Autodesk Inventor part; units mm, degrees
(part 3 of 3)
  line L680 (638.3688, 339.2047) -> (638.9016, 338.76)
  line L681 (638.9016, 338.76) -> (639.2596, 338.5571)
  line L682 (639.2596, 338.5571) -> (639.6267, 338.3665)
  line L683 (639.6267, 338.3665) -> (639.8959, 338.2197)
  line L684 (639.8959, 338.2197) -> (640.078, 338.1171)
  line L685 (640.078, 338.1171) -> (640.2676, 338.0095)
  line L686 (640.2676, 338.0095) -> (640.5028, 338.03)
  line L687 (640.5028, 338.03) -> (640.6816, 338.0539)
  line L688 (640.6816, 338.0539) -> (640.8096, 337.8945)
  line L689 (640.8096, 337.8945) -> (640.9312, 337.6444)
  line L690 (640.9312, 337.6444) -> (641.074, 337.467)
  line L691 (641.074, 337.467) -> (641.2513, 337.3173)
  line L692 (641.2513, 337.3173) -> (641.4497, 337.221)
  line L693 (641.4497, 337.221) -> (641.6459, 337.2855)
  line L694 (641.6459, 337.2855) -> (641.7783, 337.4818)
  line L695 (641.7783, 337.4818) -> (641.7901, 337.7652)
  line L696 (641.7901, 337.7652) -> (641.6541, 338.0807)
  line L697 (641.6541, 338.0807) -> (641.4196, 338.3328)
  line L698 (641.4196, 338.3328) -> (641.359, 338.4957)
  line L699 (641.359, 338.4957) -> (641.5219, 338.6755)
  line L700 (641.5219, 338.6755) -> (641.6875, 338.8527)
  line L701 (641.6875, 338.8527) -> (641.8397, 339.012)
  line L702 (641.8397, 339.012) -> (641.9195, 339.164)
  line L703 (641.9195, 339.164) -> (641.91, 339.3267)
  line L704 (641.91, 339.3267) -> (641.8249, 339.4845)
  line L705 (641.8249, 339.4845) -> (641.8179, 339.6062)
  line L706 (641.8179, 339.6062) -> (641.8756, 339.7158)
  line L707 (641.8756, 339.7158) -> (641.9948, 339.8783)
  line L708 (641.9948, 339.8783) -> (642.1243, 340.1092)
  line L709 (642.1243, 340.1092) -> (642.1842, 340.3675)
  line L710 (642.1842, 340.3675) -> (642.1632, 340.876)
  line L711 (642.1632, 340.876) -> (642.4317, 341.3803)
  line L712 (642.4317, 341.3803) -> (643.0116, 341.5945)
  line L713 (643.0116, 341.5945) -> (643.662, 341.6192)
  line L714 (643.662, 341.6192) -> (644.1803, 341.6752)
  line L715 (644.1803, 341.6752) -> (644.6825, 341.7873)
  line L716 (644.6825, 341.7873) -> (645.1009, 341.94)
  line L717 (645.1009, 341.94) -> (645.2923, 342.2013)
  line L718 (645.2923, 342.2013) -> (645.2999, 342.5311)
  line L719 (645.2999, 342.5311) -> (645.1703, 342.8111)
  line L720 (645.1703, 342.8111) -> (645.0727, 343.0529)
  line L721 (645.0727, 343.0529) -> (645.0009, 343.307)
  line L722 (645.0009, 343.307) -> (644.9495, 343.5589)
  line L723 (644.9495, 343.5589) -> (644.9292, 343.8126)
  line L724 (644.9292, 343.8126) -> (644.9075, 344.0655)
  line L725 (644.9075, 344.0655) -> (644.8528, 344.2885)
  line L726 (644.8528, 344.2885) -> (644.7662, 344.4784)
  line L727 (644.7662, 344.4784) -> (644.6518, 344.6546)
  line L728 (644.6518, 344.6546) -> (644.5158, 344.8274)
  line L729 (644.5158, 344.8274) -> (644.4573, 345.0121)
  line L730 (644.4573, 345.0121) -> (644.4937, 345.193)
  line L731 (644.4937, 345.193) -> (644.681, 345.4942)
  line L732 (644.681, 345.4942) -> (645.0696, 345.8439)
  line L733 (645.0696, 345.8439) -> (645.5473, 346.0497)
  line L734 (645.5473, 346.0497) -> (646.292, 346.1333)
  line L735 (646.292, 346.1333) -> (647.2654, 345.9804)
  line L736 (647.2654, 345.9804) -> (648.181, 345.6131)
  line L737 (648.181, 345.6131) -> (649.162, 345.0699)
  line L738 (649.162, 345.0699) -> (650.2162, 344.352)
  line L739 (650.2162, 344.352) -> (651.156, 343.4951)
  line L740 (651.156, 343.4951) -> (651.8587, 342.5889)
  line L741 (651.8587, 342.5889) -> (652.3075, 341.7803)
  line L742 (652.3075, 341.7803) -> (652.6357, 340.9186)
  line L743 (652.6357, 340.9186) -> (652.8597, 339.9664)
  line L744 (652.8597, 339.9664) -> (653.0795, 338.9452)
  line L745 (653.0795, 338.9452) -> (653.2815, 337.921)
  line L746 (653.2815, 337.921) -> (653.4749, 336.6266)
  line L747 (653.4749, 336.6266) -> (653.6329, 334.9303)
  line L748 (653.6329, 334.9303) -> (653.64, 333.2269)
  line L749 (653.64, 333.2269) -> (653.5125, 331.9053)
  line L750 (653.5125, 331.9053) -> (653.4527, 331.1762)
  line L751 (653.4527, 331.1762) -> (653.4097, 330.445)
  line L752 (653.4097, 330.445) -> (653.3768, 329.9973)
  line L753 (653.3768, 329.9973) -> (653.341, 329.9847)
  line L754 (653.341, 329.9847) -> (653.3006, 329.9705)
  line L755 (653.3006, 329.9705) -> (653.2343, 330.0785)
  line L756 (653.2343, 330.0785) -> (653.0864, 330.3682)
  line L757 (653.0864, 330.3682) -> (652.9397, 330.6585)
  line L758 (652.9397, 330.6585) -> (652.5578, 331.4365)
  line L759 (652.5578, 331.4365) -> (651.7302, 332.977)
  line L760 (651.7302, 332.977) -> (650.7272, 334.4004)
  line L761 (650.7272, 334.4004) -> (649.6787, 335.4361)
  line L762 (649.6787, 335.4361) -> (648.9013, 336.0163)
  line L763 (648.9013, 336.0163) -> (648.0503, 336.4816)
  line L764 (648.0503, 336.4816) -> (647.2286, 336.7737)
  line L765 (647.2286, 336.7737) -> (646.5919, 336.9521)
  line L766 (646.5919, 336.9521) -> (645.9486, 337.0788)
  line L767 (645.9486, 337.0788) -> (645.3737, 337.118)
  line L768 (645.3737, 337.118) -> (644.935, 337.0846)
  line L769 (644.935, 337.0846) -> (644.4965, 337.0158)
  line L770 (644.4965, 337.0158) -> (644.0896, 336.9396)
  line L771 (644.0896, 336.9396) -> (643.7371, 336.8506)
  line L772 (643.7371, 336.8506) -> (643.3867, 336.7494)
  line L773 (643.3867, 336.7494) -> (642.9684, 336.6283)
  line L774 (642.9684, 336.6283) -> (642.4606, 336.4025)
  line L775 (642.4606, 336.4025) -> (641.9974, 336.1008)
  line L776 (641.9974, 336.1008) -> (641.4154, 335.5958)
  line L777 (641.4154, 335.5958) -> (640.6559, 334.7195)
  line L778 (640.6559, 334.7195) -> (640.0496, 333.7342)
  line L779 (640.0496, 333.7342) -> (639.598, 332.6628)
  line L780 (639.598, 332.6628) -> (639.4033, 331.5928)
  line L781 (639.4033, 331.5928) -> (639.5285, 330.5297)
  line L782 (639.5285, 330.5297) -> (639.9163, 329.6261)
  line L783 (639.9163, 329.6261) -> (640.2591, 329.0578)
  line L784 (640.2591, 329.0578) -> (640.7016, 328.5777)
  line L785 (640.7016, 328.5777) -> (641.3259, 328.2297)
  line L786 (641.3259, 328.2297) -> (642.0543, 327.9898)
  line L787 (642.0543, 327.9898) -> (642.8045, 327.9153)
  line L788 (642.8045, 327.9153) -> (643.4239, 328.0198)
  line L789 (643.4239, 328.0198) -> (643.7234, 328.164)
  line L790 (643.7234, 328.164) -> (644.0036, 328.3597)
  line L791 (644.0036, 328.3597) -> (644.2303, 328.545)
  line L792 (644.2303, 328.545) -> (644.3579, 328.5949)
  line L793 (644.3579, 328.5949) -> (644.4647, 328.5515)
  line L794 (644.4647, 328.5515) -> (644.6078, 328.5483)
  line L795 (644.6078, 328.5483) -> (644.8137, 328.7622)
  line L796 (644.8137, 328.7622) -> (645.0075, 328.9633)
  line L797 (645.0075, 328.9633) -> (645.2007, 329.0779)
  line L798 (645.2007, 329.0779) -> (645.4102, 329.0354)
  line L799 (645.4102, 329.0354) -> (645.6024, 328.9962)
  line L800 (645.6024, 328.9962) -> (645.775, 329.1124)
  line L801 (645.775, 329.1124) -> (645.9143, 329.5669)
  line L802 (645.9143, 329.5669) -> (646.0494, 330.0046)
  line L803 (646.0494, 330.0046) -> (646.1598, 330.3696)
  line L804 (646.1598, 330.3696) -> (646.1419, 330.5458)
  line L805 (646.1419, 330.5458) -> (646.04, 330.6792)
  line L806 (646.04, 330.6792) -> (645.7833, 330.864)
  line L807 (645.7833, 330.864) -> (645.4962, 331.381)
  line L808 (645.4962, 331.381) -> (645.5693, 331.9567)
  line L809 (645.5693, 331.9567) -> (645.9469, 332.3437)
  line L810 (645.9469, 332.3437) -> (646.3957, 332.4185)
  line L811 (646.3957, 332.4185) -> (646.8578, 332.3259)
  line L812 (646.8578, 332.3259) -> (647.1637, 332.0494)
  line L813 (647.1637, 332.0494) -> (647.2902, 331.5479)
  line L814 (647.2902, 331.5479) -> (647.1838, 331.048)
  line L815 (647.1838, 331.048) -> (646.9158, 330.7499)
  line L816 (646.9158, 330.7499) -> (646.8237, 330.6249)
  line L817 (646.8237, 330.6249) -> (646.8245, 330.496)
  line L818 (646.8245, 330.496) -> (646.909, 330.2956)
  line L819 (646.909, 330.2956) -> (647.078, 329.9354)
  line L820 (647.078, 329.9354) -> (647.2514, 329.5773)
  line L821 (647.2514, 329.5773) -> (647.4089, 329.2696)
  line L822 (647.4089, 329.2696) -> (647.5223, 329.1487)
  line L823 (647.5223, 329.1487) -> (647.6603, 329.1508)
  line L824 (647.6603, 329.1508) -> (647.8084, 329.2959)
  line L825 (647.8084, 329.2959) -> (647.9268, 329.3852)
  line L826 (647.9268, 329.3852) -> (648.0544, 329.3725)
  line L827 (648.0544, 329.3725) -> (648.1713, 329.2651)
  line L828 (648.1713, 329.2651) -> (648.2406, 329.2248)
  line L829 (648.2406, 329.2248) -> (648.3206, 329.1923)
  line L830 (648.3206, 329.1923) -> (648.4374, 329.1145)
  line L831 (648.4374, 329.1145) -> (648.6695, 329.026)
  line L832 (648.6695, 329.026) -> (648.8857, 329.0926)
  line L833 (648.8857, 329.0926) -> (649.1375, 329.3402)
  line L834 (649.1375, 329.3402) -> (649.338, 329.6124)
  line L835 (649.338, 329.6124) -> (649.2845, 329.8203)
  line L836 (649.2845, 329.8203) -> (648.9894, 330.1015)
  line L837 (648.9894, 330.1015) -> (648.8461, 330.3743)
  line L838 (648.8461, 330.3743) -> (648.8467, 330.6597)
  line L839 (648.8467, 330.6597) -> (648.9019, 330.9534)
  line L840 (648.9019, 330.9534) -> (649.0437, 331.1526)
  line L841 (649.0437, 331.1526) -> (649.2599, 331.256)
  line L842 (649.2599, 331.256) -> (649.5081, 331.3325)
  line L843 (649.5081, 331.3325) -> (649.7429, 331.4624)
  line L844 (649.7429, 331.4624) -> (649.8689, 331.644)
  line L845 (649.8689, 331.644) -> (649.8709, 331.9244)
  line L846 (649.8709, 331.9244) -> (649.7689, 332.2531)
  line L847 (649.7689, 332.2531) -> (649.5634, 332.4074)
  line L848 (649.5634, 332.4074) -> (649.1862, 332.4392)
  line L849 (649.1862, 332.4392) -> (648.8348, 332.4703)
  line L850 (648.8348, 332.4703) -> (648.6591, 332.6342)
  line L851 (648.6591, 332.6342) -> (648.5396, 332.9759)
  line L852 (648.5396, 332.9759) -> (648.5396, 333.1972)
  line L853 (648.5396, 333.1972) -> (648.5993, 333.4307)
  line L854 (648.5993, 333.4307) -> (648.6908, 333.6545)
  line L855 (648.6908, 333.6545) -> (648.7603, 333.8764)
  line L856 (648.7603, 333.8764) -> (648.7114, 334.0594)
  line L857 (648.7114, 334.0594) -> (648.5368, 334.1793)
  line L858 (648.5368, 334.1793) -> (648.5255, 334.1971)
  line L859 (648.5255, 334.1971) -> (648.4352, 334.2619)
  line L860 (648.4352, 334.2619) -> (648.1296, 334.43)
  line L861 (648.1296, 334.43) -> (647.8956, 334.3619)
  line L862 (647.8956, 334.3619) -> (647.5624, 334.0726)
  line L863 (647.5624, 334.0726) -> (647.1848, 333.9698)
  line L864 (647.1848, 333.9698) -> (646.8096, 334.0976)
  line L865 (646.8096, 334.0976) -> (646.6055, 334.3548)
  line L866 (646.6055, 334.3548) -> (646.5912, 334.3837)
  line L867 (646.5912, 334.3837) -> (646.5764, 334.4123)
  line L868 (646.5764, 334.4123) -> (646.5328, 334.5402)
  line L869 (646.5328, 334.5402) -> (646.36, 334.9153)
  line L870 (646.36, 334.9153) -> (646.1032, 335.0114)
  line L871 (646.1032, 335.0114) -> (645.6643, 334.9395)
  line L872 (645.6643, 334.9395) -> (645.4263, 334.8369)
  line L873 (645.4263, 334.8369) -> (645.3011, 334.6517)
  line L874 (645.3011, 334.6517) -> (645.2925, 334.3663)
  line L875 (645.2925, 334.3663) -> (645.3093, 334.0823)
  line L876 (645.3093, 334.0823) -> (645.2219, 333.8429)
  line L877 (645.2219, 333.8429) -> (644.945, 333.7417)
  line L878 (644.945, 333.7417) -> (644.6953, 333.7646)
  line L879 (644.6953, 333.7646) -> (644.4442, 333.8373)
  line L880 (644.4442, 333.8373) -> (644.2089, 333.9335)
  line L881 (644.2089, 333.9335) -> (644.0187, 333.9855)
  line L882 (644.0187, 333.9855) -> (643.8593, 333.9464)
  line L883 (643.8593, 333.9464) -> (643.7235, 333.7943)
  line L884 (643.7235, 333.7943) -> (643.6129, 333.639)
  line L885 (643.6129, 333.639) -> (643.5021, 333.4846)
  line L886 (643.5021, 333.4846) -> (643.4129, 333.3388)
  line L887 (643.4129, 333.3388) -> (643.4033, 333.2638)
  line L888 (643.4033, 333.2638) -> (643.4201, 333.1782)
  line L889 (643.4201, 333.1782) -> (643.4548, 333.1005)
  line L890 (643.4548, 333.1005) -> (643.5125, 333.014)
  line L891 (643.5125, 333.014) -> (643.5832, 332.9366)
  line L892 (643.5832, 332.9366) -> (643.6908, 332.8603)
  line L893 (643.6908, 332.8603) -> (643.873, 332.6566)
  line L894 (643.873, 332.6566) -> (643.9145, 332.4144)
  line L895 (643.9145, 332.4144) -> (643.8537, 332.1496)
  line L896 (643.8537, 332.1496) -> (643.707, 331.9584)
  line L897 (643.707, 331.9584) -> (643.4973, 331.8541)
  line L898 (643.4973, 331.8541) -> (643.2471, 331.7944)
  line L899 (643.2471, 331.7944) -> (642.9748, 331.7079)
  line L900 (642.9748, 331.7079) -> (642.8635, 331.5446)
  line L901 (642.8635, 331.5446) -> (642.8564, 331.2503)
  line L902 (642.8564, 331.2503) -> (642.8748, 331.0939)
  line L903 (642.8748, 331.0939) -> (642.9069, 330.9388)
  line L904 (642.9069, 330.9388) -> (642.9519, 330.7854)
  line L905 (642.9519, 330.7854) -> (643.0305, 330.6385)
  line L906 (643.0305, 330.6385) -> (643.157, 330.5503)
  line L907 (643.157, 330.5503) -> (643.3332, 330.5435)
  line L908 (643.3332, 330.5435) -> (643.4393, 330.5501)
  line L909 (643.4393, 330.5501) -> (643.5468, 330.5473)
  line L910 (643.5468, 330.5473) -> (643.6532, 330.5448)
  line L911 (643.6532, 330.5448) -> (643.7491, 330.5448)
  line L912 (643.7491, 330.5448) -> (643.8447, 330.5448)
  line L913 (643.8447, 330.5448) -> (643.9373, 330.5335)
  line L914 (643.9373, 330.5335) -> (644.0077, 330.4198)
  line L915 (644.0077, 330.4198) -> (644.0762, 330.3087)
  line L916 (644.0762, 330.3087) -> (644.145, 330.1957)
  line L917 (644.145, 330.1957) -> (644.2082, 330.0593)
  line L918 (644.2082, 330.0593) -> (644.2134, 329.9194)
  line L919 (644.2134, 329.9194) -> (644.1345, 329.7525)
  line L920 (644.1345, 329.7525) -> (644.0315, 329.5229)
  line L921 (644.0315, 329.5229) -> (643.9541, 329.2758)
  line L922 (643.9541, 329.2758) -> (643.8606, 329.0458)
  line L923 (643.8606, 329.0458) -> (643.7682, 328.9163)
  line L924 (643.7682, 328.9163) -> (643.648, 328.8027)
  line L925 (643.648, 328.8027) -> (643.4908, 328.6975)
  line L926 (643.4908, 328.6975) -> (643.0298, 328.517)
  line L927 (643.0298, 328.517) -> (642.5469, 328.4669)
  line L928 (642.5469, 328.4669) -> (641.9833, 328.5284)
  line L929 (641.9833, 328.5284) -> (640.9886, 328.9796)
  line L930 (640.9886, 328.9796) -> (640.4, 329.7751)
  line L931 (640.4, 329.7751) -> (640.0785, 330.8118)
  line L932 (640.0785, 330.8118) -> (640.0376, 331.8559)
  line L933 (640.0376, 331.8559) -> (640.2756, 332.8422)
  line L934 (640.2756, 332.8422) -> (640.6932, 333.7772)
  line L935 (640.6932, 333.7772) -> (641.1525, 334.5329)
  line L936 (641.1525, 334.5329) -> (641.7257, 335.1987)
  line L937 (641.7257, 335.1987) -> (642.4244, 335.7328)
  line L938 (642.4244, 335.7328) -> (642.896, 335.9865)
  line L939 (642.896, 335.9865) -> (643.3858, 336.1925)
  line L940 (643.3858, 336.1925) -> (643.9119, 336.3603)
  line L941 (643.9119, 336.3603) -> (644.7048, 336.4976)
  line L942 (644.7048, 336.4976) -> (645.4965, 336.5084)
  line L943 (645.4965, 336.5084) -> (646.3068, 336.4278)
  line L944 (646.3068, 336.4278) -> (647.6933, 336.056)
  line L945 (647.6933, 336.056) -> (648.9249, 335.3691)
  line L946 (648.9249, 335.3691) -> (649.987, 334.3777)
  line L947 (649.987, 334.3777) -> (650.8539, 333.2703)
  line L948 (650.8539, 333.2703) -> (651.5929, 332.0841)
  line L949 (651.5929, 332.0841) -> (652.1726, 330.8305)
  line L950 (652.1726, 330.8305) -> (652.3954, 330.1499)
  line L951 (652.3954, 330.1499) -> (652.5787, 329.4541)
  line L952 (652.5787, 329.4541) -> (652.756, 328.7737)
  line L953 (652.756, 328.7737) -> (652.7913, 328.6615)
  line L954 (652.7913, 328.6615) -> (652.8256, 328.5492)
  line L955 (652.8256, 328.5492) -> (652.846, 328.4355)
  line L956 (652.846, 328.4355) -> (652.8488, 328.3155)
  line L957 (652.8488, 328.3155) -> (652.8379, 328.1947)
  line L958 (652.8379, 328.1947) -> (652.8126, 328.0728)
  line L959 (652.8126, 328.0728) -> (652.7004, 327.7128)
  line L960 (652.7004, 327.7128) -> (652.587, 327.3536)
  line L961 (652.587, 327.3536) -> (652.5137, 326.989)
  line L962 (652.5137, 326.989) -> (652.4875, 326.5028)
  line L963 (652.4875, 326.5028) -> (652.4932, 326.0162)
  line L964 (652.4932, 326.0162) -> (652.497, 325.5388)
  line L965 (652.497, 325.5388) -> (651.6782, 325.6846)
  line L966 (651.6782, 325.6846) -> (650.8654, 325.8294)
  line L967 (650.8654, 325.8294) -> (650.0544, 325.974)
  line L968 (650.0544, 325.974) -> (649.8801, 325.994)
  line L969 (649.8801, 325.994) -> (649.6801, 325.9973)
  line L970 (649.6801, 325.9973) -> (649.5362, 325.9926)
  line L971 (649.5362, 325.9926) -> (649.4314, 326.0058)
  line L972 (649.4314, 326.0058) -> (649.3484, 326.0632)
  line L973 (649.3484, 326.0632) -> (649.1744, 326.2849)
  line L974 (649.1744, 326.2849) -> (649.0251, 326.5004)
  line L975 (649.0251, 326.5004) -> (648.8782, 326.6945)
  line L976 (648.8782, 326.6945) -> (648.7116, 326.8518)
  line L977 (648.7116, 326.8518) -> (648.503, 326.957)
  line L978 (648.503, 326.957) -> (648.0715, 327.0815)
  line L979 (648.0715, 327.0815) -> (647.6351, 327.1908)
  line L980 (647.6351, 327.1908) -> (647.1955, 327.2898)
  line L981 (647.1955, 327.2898) -> (646.7543, 327.3832)
  line L982 (646.7543, 327.3832) -> (646.3134, 327.4759)
  line L983 (646.3134, 327.4759) -> (646.2424, 327.4827)
  line L984 (646.2424, 327.4827) -> (646.1643, 327.4758)
  line L985 (646.1643, 327.4758) -> (646.0874, 327.4565)
  line L986 (646.0874, 327.4565) -> (646.0201, 327.426)
  line L987 (646.0201, 327.426) -> (645.9709, 327.3853)
  line L988 (645.9709, 327.3853) -> (645.9488, 327.3349)
  line L989 (645.9488, 327.3349) -> (645.9434, 327.2662)
  line L990 (645.9434, 327.2662) -> (645.9522, 327.189)
  line L991 (645.9522, 327.189) -> (645.9723, 327.113)
  line L992 (645.9723, 327.113) -> (646.0012, 327.0481)
  line L993 (646.0012, 327.0481) -> (646.2363, 326.6383)
  line L994 (646.2363, 326.6383) -> (646.4739, 326.2298)
  line L995 (646.4739, 326.2298) -> (646.714, 325.8229)
  line L996 (646.714, 325.8229) -> (646.9568, 325.4176)
  line L997 (646.9568, 325.4176) -> (647.2027, 325.0142)
  line L998 (647.2027, 325.0142) -> (647.2664, 324.9233)
  line L999 (647.2664, 324.9233) -> (647.34, 324.8379)
  line L1000 (647.34, 324.8379) -> (647.4204, 324.757)
  line L1001 (647.4204, 324.757) -> (647.5045, 324.6793)
  line L1002 (647.5045, 324.6793) -> (647.5891, 324.6038)
  line L1003 (647.5891, 324.6038) -> (647.7055, 324.5163)
  line L1004 (647.7055, 324.5163) -> (647.8242, 324.463)
  line L1005 (647.8242, 324.463) -> (647.9492, 324.447)
  line L1006 (647.9492, 324.447) -> (648.0846, 324.4712)
  line L1007 (648.0846, 324.4712) -> (648.2342, 324.5385)
  line L1008 (648.2342, 324.5385) -> (648.6906, 324.7631)
  line L1009 (648.6906, 324.7631) -> (649.1634, 324.928)
  line L1010 (649.1634, 324.928) -> (649.6497, 325.0333)
  line L1011 (649.6497, 325.0333) -> (650.1465, 325.079)
  line L1012 (650.1465, 325.079) -> (650.6512, 325.0647)
  line L1013 (650.6512, 325.0647) -> (650.9264, 325.0335)
  line L1014 (650.9264, 325.0335) -> (651.2001, 324.9759)
  line L1015 (651.2001, 324.9759) -> (651.4581, 324.8744)
  line L1016 (651.4581, 324.8744) -> (651.6862, 324.7113)
  line L1017 (651.6862, 324.7113) -> (651.8704, 324.4692)
  line L1018 (651.8704, 324.4692) -> (651.9281, 324.3641)
  line L1019 (651.9281, 324.3641) -> (651.9845, 324.2555)
  line L1020 (651.9845, 324.2555) -> (652.033, 324.1447)
  line L1021 (652.033, 324.1447) -> (652.0672, 324.0332)
  line L1022 (652.0672, 324.0332) -> (652.0809, 323.9222)
  line L1023 (652.0809, 323.9222) -> (652.0815, 323.5641)
  line L1024 (652.0815, 323.5641) -> (652.0753, 323.2056)
  line L1025 (652.0753, 323.2056) -> (652.0626, 322.8472)
  line L1026 (652.0626, 322.8472) -> (652.0437, 322.4892)
  line L1027 (652.0437, 322.4892) -> (652.019, 322.1317)
  line L1028 (652.019, 322.1317) -> (651.9957, 321.8513)
  line L1029 (651.9957, 321.8513) -> (651.9676, 321.5703)
  line L1030 (651.9676, 321.5703) -> (651.931, 321.2906)
  line L1031 (651.931, 321.2906) -> (651.8825, 321.0137)
  line L1032 (651.8825, 321.0137) -> (651.8184, 320.7414)
  line L1033 (651.8184, 320.7414) -> (651.6906, 320.326)
  line L1034 (651.6906, 320.326) -> (651.5301, 319.9279)
  line L1035 (651.5301, 319.9279) -> (651.3279, 319.5501)
  line L1036 (651.3279, 319.5501) -> (651.0746, 319.1952)
  line L1037 (651.0746, 319.1952) -> (650.7612, 318.8663)
  line L1038 (650.7612, 318.8663) -> (650.1765, 318.3235)
  line L1039 (650.1765, 318.3235) -> (649.6021, 317.7693)
  line L1040 (649.6021, 317.7693) -> (649.0366, 317.2058)
  line L1041 (649.0366, 317.2058) -> (648.4786, 316.6348)
  line L1042 (648.4786, 316.6348) -> (647.9268, 316.0583)
  line L1043 (647.9268, 316.0583) -> (647.4527, 315.513)
  line L1044 (647.4527, 315.513) -> (647.0352, 314.931)
  line L1045 (647.0352, 314.931) -> (646.6822, 314.3123)
  line L1046 (646.6822, 314.3123) -> (646.4012, 313.6567)
  line L1047 (646.4012, 313.6567) -> (646.2001, 312.964)
  line L1048 (646.2001, 312.964) -> (646.1012, 312.4781)
  line L1049 (646.1012, 312.4781) -> (646.0225, 311.9852)
  line L1050 (646.0225, 311.9852) -> (645.9687, 311.4888)
  line L1051 (645.9687, 311.4888) -> (645.9446, 310.9925)
  line L1052 (645.9446, 310.9925) -> (645.9547, 310.5002)
  line L1053 (645.9547, 310.5002) -> (646.0213, 309.8862)
  line L1054 (646.0213, 309.8862) -> (646.1473, 309.2827)
  line L1055 (646.1473, 309.2827) -> (646.3314, 308.6926)
  line L1056 (646.3314, 308.6926) -> (646.5721, 308.119)
  line L1057 (646.5721, 308.119) -> (646.8679, 307.565)
  line L1058 (646.8679, 307.565) -> (647.2492, 306.9543)
  line L1059 (647.2492, 306.9543) -> (647.6667, 306.3618)
  line L1060 (647.6667, 306.3618) -> (648.1265, 305.8027)
  line L1061 (648.1265, 305.8027) -> (648.6347, 305.2921)
  line L1062 (648.6347, 305.2921) -> (649.1975, 304.8453)
  line L1063 (649.1975, 304.8453) -> (631.0701, 305.6803)
  line L1064 (631.0701, 305.6803) -> (587.8432, 307.6714)
  line L1065 (587.8432, 307.6714) -> (536.2498, 310.0479)
  line L1066 (536.2498, 310.0479) -> (493.0229, 312.039)
  line L1067 (493.0229, 312.039) -> (436.4362, 314.6455)
  line L1068 (436.4362, 314.6455) -> (416.3257, 317.8792)
  line L1069 (416.3257, 317.8792) -> (164.2007, 302.4811)
  line L1070 (164.2007, 302.4811) -> (35.8306, 311.154)
  point P0 (-87.4375, 600)
  constraints: 2142 end point
sketch "Sketch3" plane through (87.4375, 600, -660) normal (0, 0, 1) x (1, 0, 0)
  line L0 (48.6601, -423.7213) -> (48.4084, -423.1135) projected
  line L1 (48.4084, -423.1135) -> (48.3225, -422.4613) projected
  line L2 (48.3225, -422.4613) -> (48.4084, -421.8091) projected
  line L3 (48.4084, -421.8091) -> (48.6601, -421.2013) projected
  line L4 (48.6601, -421.2013) -> (49.0606, -420.6794) projected
  line L5 (49.0606, -420.6794) -> (49.5825, -420.2789) projected
  line L6 (49.5825, -420.2789) -> (50.1903, -420.0271) projected
  line L7 (50.1903, -420.0271) -> (50.8425, -419.9413) projected
  line L8 (50.8425, -419.9413) -> (51.4947, -420.0271) projected
  line L9 (51.4947, -420.0271) -> (52.1025, -420.2789) projected
  line L10 (52.1025, -420.2789) -> (52.6244, -420.6794) projected
  line L11 (52.6244, -420.6794) -> (53.0249, -421.2013) projected
  line L12 (53.0249, -421.2013) -> (53.2766, -421.8091) projected
  line L13 (53.2766, -421.8091) -> (53.3625, -422.4613) projected
  line L14 (53.3625, -422.4613) -> (53.2766, -423.1135) projected
  line L15 (53.2766, -423.1135) -> (53.0249, -423.7213) projected
  line L16 (53.0249, -423.7213) -> (52.6244, -424.2432) projected
  line L17 (52.6244, -424.2432) -> (52.1025, -424.6437) projected
  line L18 (52.1025, -424.6437) -> (51.4947, -424.8954) projected
  line L19 (51.4947, -424.8954) -> (50.8425, -424.9813) projected
  line L20 (50.8425, -424.9813) -> (50.1903, -424.8954) projected
  line L21 (50.1903, -424.8954) -> (49.5825, -424.6437) projected
  line L22 (49.5825, -424.6437) -> (49.0606, -424.2432) projected
  line L23 (49.0606, -424.2432) -> (48.6601, -423.7213) projected
  line L24 (236.8925, -369.9813) -> (236.2403, -369.8954) projected
  line L25 (236.2403, -369.8954) -> (235.6325, -369.6437) projected
  line L26 (235.6325, -369.6437) -> (235.1106, -369.2432) projected
  line L27 (235.1106, -369.2432) -> (234.7101, -368.7213) projected
  line L28 (234.7101, -368.7213) -> (234.4584, -368.1135) projected
  line L29 (234.4584, -368.1135) -> (234.3725, -367.4613) projected
  line L30 (234.3725, -367.4613) -> (234.4584, -366.8091) projected
  line L31 (234.4584, -366.8091) -> (234.7101, -366.2013) projected
  line L32 (234.7101, -366.2013) -> (235.1106, -365.6794) projected
  line L33 (235.1106, -365.6794) -> (235.6325, -365.2789) projected
  line L34 (235.6325, -365.2789) -> (236.2403, -365.0271) projected
  line L35 (236.2403, -365.0271) -> (236.8925, -364.9413) projected
  line L36 (236.8925, -364.9413) -> (237.5447, -365.0271) projected
  line L37 (237.5447, -365.0271) -> (238.1525, -365.2789) projected
  line L38 (238.1525, -365.2789) -> (238.6744, -365.6794) projected
  line L39 (238.6744, -365.6794) -> (239.0749, -366.2013) projected
  line L40 (239.0749, -366.2013) -> (239.3266, -366.8091) projected
  line L41 (239.3266, -366.8091) -> (239.4125, -367.4613) projected
  line L42 (239.4125, -367.4613) -> (239.3266, -368.1135) projected
  line L43 (239.3266, -368.1135) -> (239.0749, -368.7213) projected
  line L44 (239.0749, -368.7213) -> (238.6744, -369.2432) projected
  line L45 (238.6744, -369.2432) -> (238.1525, -369.6437) projected
  line L46 (238.1525, -369.6437) -> (237.5447, -369.8954) projected
  line L47 (237.5447, -369.8954) -> (236.8925, -369.9813) projected
  line L48 (234.4584, -298.1135) -> (234.3725, -297.4613) projected
  line L49 (234.3725, -297.4613) -> (234.4584, -296.809) projected
  line L50 (234.4584, -296.809) -> (234.7101, -296.2012) projected
  line L51 (234.7101, -296.2012) -> (235.1106, -295.6793) projected
  line L52 (235.1106, -295.6793) -> (235.6325, -295.2789) projected
  line L53 (235.6325, -295.2789) -> (236.2403, -295.0271) projected
  line L54 (236.2403, -295.0271) -> (236.8925, -294.9413) projected
  line L55 (236.8925, -294.9413) -> (237.5447, -295.0271) projected
  line L56 (237.5447, -295.0271) -> (238.1525, -295.2789) projected
  line L57 (238.1525, -295.2789) -> (238.6744, -295.6793) projected
  line L58 (238.6744, -295.6793) -> (239.0749, -296.2012) projected
  line L59 (239.0749, -296.2012) -> (239.3266, -296.809) projected
  line L60 (239.3266, -296.809) -> (239.4125, -297.4613) projected
  line L61 (239.4125, -297.4613) -> (239.3266, -298.1135) projected
  line L62 (239.3266, -298.1135) -> (239.0749, -298.7212) projected
  line L63 (239.0749, -298.7212) -> (238.6744, -299.2432) projected
  line L64 (238.6744, -299.2432) -> (238.1525, -299.6437) projected
  line L65 (238.1525, -299.6437) -> (237.5447, -299.8954) projected
  line L66 (237.5447, -299.8954) -> (236.8925, -299.9813) projected
  line L67 (236.8925, -299.9813) -> (236.2403, -299.8954) projected
  line L68 (236.2403, -299.8954) -> (235.6325, -299.6437) projected
  line L69 (235.6325, -299.6437) -> (235.1106, -299.2432) projected
  line L70 (235.1106, -299.2432) -> (234.7101, -298.7212) projected
  line L71 (234.7101, -298.7212) -> (234.4584, -298.1135) projected
  line L72 (48.6601, -368.7213) -> (48.4084, -368.1135) projected
  line L73 (48.4084, -368.1135) -> (48.3225, -367.4613) projected
  line L74 (48.3225, -367.4613) -> (48.4084, -366.8091) projected
  line L75 (48.4084, -366.8091) -> (48.6601, -366.2013) projected
  line L76 (48.6601, -366.2013) -> (49.0606, -365.6794) projected
  line L77 (49.0606, -365.6794) -> (49.5825, -365.2789) projected
  line L78 (49.5825, -365.2789) -> (50.1903, -365.0271) projected
  line L79 (50.1903, -365.0271) -> (50.8425, -364.9413) projected
  line L80 (50.8425, -364.9413) -> (51.4947, -365.0271) projected
  line L81 (51.4947, -365.0271) -> (52.1025, -365.2789) projected
  line L82 (52.1025, -365.2789) -> (52.6244, -365.6794) projected
  line L83 (52.6244, -365.6794) -> (53.0249, -366.2013) projected
  line L84 (53.0249, -366.2013) -> (53.2766, -366.8091) projected
  line L85 (53.2766, -366.8091) -> (53.3625, -367.4613) projected
  line L86 (53.3625, -367.4613) -> (53.2766, -368.1135) projected
  line L87 (53.2766, -368.1135) -> (53.0249, -368.7213) projected
  line L88 (53.0249, -368.7213) -> (52.6244, -369.2432) projected
  line L89 (52.6244, -369.2432) -> (52.1025, -369.6437) projected
  line L90 (52.1025, -369.6437) -> (51.4947, -369.8954) projected
  line L91 (51.4947, -369.8954) -> (50.8425, -369.9813) projected
  line L92 (50.8425, -369.9813) -> (50.1903, -369.8954) projected
  line L93 (50.1903, -369.8954) -> (49.5825, -369.6437) projected
  line L94 (49.5825, -369.6437) -> (49.0606, -369.2432) projected
  line L95 (49.0606, -369.2432) -> (48.6601, -368.7213) projected
  line L96 (48.6601, -298.7212) -> (48.4084, -298.1135) projected
  line L97 (48.4084, -298.1135) -> (48.3225, -297.4613) projected
  line L98 (48.3225, -297.4613) -> (48.4084, -296.809) projected
  line L99 (48.4084, -296.809) -> (48.6601, -296.2012) projected
  line L100 (48.6601, -296.2012) -> (49.0606, -295.6793) projected
  line L101 (49.0606, -295.6793) -> (49.5825, -295.2789) projected
  line L102 (49.5825, -295.2789) -> (50.1903, -295.0271) projected
  line L103 (50.1903, -295.0271) -> (50.8425, -294.9413) projected
  line L104 (50.8425, -294.9413) -> (51.4947, -295.0271) projected
  line L105 (51.4947, -295.0271) -> (52.1025, -295.2789) projected
  line L106 (52.1025, -295.2789) -> (52.6244, -295.6793) projected
  line L107 (52.6244, -295.6793) -> (53.0249, -296.2012) projected
  line L108 (53.0249, -296.2012) -> (53.2766, -296.809) projected
  line L109 (53.2766, -296.809) -> (53.3625, -297.4613) projected
  line L110 (53.3625, -297.4613) -> (53.2766, -298.1135) projected
  line L111 (53.2766, -298.1135) -> (53.0249, -298.7212) projected
  line L112 (53.0249, -298.7212) -> (52.6244, -299.2432) projected
  line L113 (52.6244, -299.2432) -> (52.1025, -299.6437) projected
  line L114 (52.1025, -299.6437) -> (51.4947, -299.8954) projected
  line L115 (51.4947, -299.8954) -> (50.8425, -299.9813) projected
  line L116 (50.8425, -299.9813) -> (50.1903, -299.8954) projected
  line L117 (50.1903, -299.8954) -> (49.5825, -299.6437) projected
  line L118 (49.5825, -299.6437) -> (49.0606, -299.2432) projected
  line L119 (49.0606, -299.2432) -> (48.6601, -298.7212) projected
  line L120 (492.6101, -368.7213) -> (492.3584, -368.1135) projected
  line L121 (492.3584, -368.1135) -> (492.2725, -367.4613) projected
  line L122 (492.2725, -367.4613) -> (492.3584, -366.8091) projected
  line L123 (492.3584, -366.8091) -> (492.6101, -366.2013) projected
  line L124 (492.6101, -366.2013) -> (493.0106, -365.6794) projected
  line L125 (493.0106, -365.6794) -> (493.5325, -365.2789) projected
  line L126 (493.5325, -365.2789) -> (494.1403, -365.0271) projected
  line L127 (494.1403, -365.0271) -> (494.7925, -364.9413) projected
  line L128 (494.7925, -364.9413) -> (495.4447, -365.0271) projected
  line L129 (495.4447, -365.0271) -> (496.0525, -365.2789) projected
  line L130 (496.0525, -365.2789) -> (496.5744, -365.6794) projected
  line L131 (496.5744, -365.6794) -> (496.9749, -366.2013) projected
  line L132 (496.9749, -366.2013) -> (497.2266, -366.8091) projected
  line L133 (497.2266, -366.8091) -> (497.3125, -367.4613) projected
  line L134 (497.3125, -367.4613) -> (497.2266, -368.1135) projected
  line L135 (497.2266, -368.1135) -> (496.9749, -368.7213) projected
  line L136 (496.9749, -368.7213) -> (496.5744, -369.2432) projected
  line L137 (496.5744, -369.2432) -> (496.0525, -369.6437) projected
  line L138 (496.0525, -369.6437) -> (495.4447, -369.8954) projected
  line L139 (495.4447, -369.8954) -> (494.7925, -369.9813) projected
  line L140 (494.7925, -369.9813) -> (494.1403, -369.8954) projected
  line L141 (494.1403, -369.8954) -> (493.5325, -369.6437) projected
  line L142 (493.5325, -369.6437) -> (493.0106, -369.2432) projected
  line L143 (493.0106, -369.2432) -> (492.6101, -368.7213) projected
  line L144 (492.6101, -298.7212) -> (492.3584, -298.1135) projected
  line L145 (492.3584, -298.1135) -> (492.2725, -297.4613) projected
  line L146 (492.2725, -297.4613) -> (492.3584, -296.809) projected
  line L147 (492.3584, -296.809) -> (492.6101, -296.2012) projected
  line L148 (492.6101, -296.2012) -> (493.0106, -295.6793) projected
  line L149 (493.0106, -295.6793) -> (493.5325, -295.2789) projected
  line L150 (493.5325, -295.2789) -> (494.1403, -295.0271) projected
  line L151 (494.1403, -295.0271) -> (494.7925, -294.9413) projected
  line L152 (494.7925, -294.9413) -> (495.4447, -295.0271) projected
  line L153 (495.4447, -295.0271) -> (496.0525, -295.2789) projected
  line L154 (496.0525, -295.2789) -> (496.5744, -295.6793) projected
  line L155 (496.5744, -295.6793) -> (496.9749, -296.2012) projected
  line L156 (496.9749, -296.2012) -> (497.2266, -296.809) projected
  line L157 (497.2266, -296.809) -> (497.3125, -297.4613) projected
  line L158 (497.3125, -297.4613) -> (497.2266, -298.1135) projected
  line L159 (497.2266, -298.1135) -> (496.9749, -298.7212) projected
  line L160 (496.9749, -298.7212) -> (496.5744, -299.2432) projected
  line L161 (496.5744, -299.2432) -> (496.0525, -299.6437) projected
  line L162 (496.0525, -299.6437) -> (495.4447, -299.8954) projected
  line L163 (495.4447, -299.8954) -> (494.7925, -299.9813) projected
  line L164 (494.7925, -299.9813) -> (494.1403, -299.8954) projected
  line L165 (494.1403, -299.8954) -> (493.5325, -299.6437) projected
  line L166 (493.5325, -299.6437) -> (493.0106, -299.2432) projected
  line L167 (493.0106, -299.2432) -> (492.6101, -298.7212) projected
  line L168 (105.1903, -369.8954) -> (104.5825, -369.6437) projected
  line L169 (104.5825, -369.6437) -> (104.0606, -369.2432) projected
  line L170 (104.0606, -369.2432) -> (103.6601, -368.7213) projected
  line L171 (103.6601, -368.7213) -> (103.4084, -368.1135) projected
  line L172 (103.4084, -368.1135) -> (103.3225, -367.4613) projected
  line L173 (103.3225, -367.4613) -> (103.4084, -366.8091) projected
  line L174 (103.4084, -366.8091) -> (103.6601, -366.2013) projected
  line L175 (103.6601, -366.2013) -> (104.0606, -365.6794) projected
  line L176 (104.0606, -365.6794) -> (104.5825, -365.2789) projected
  line L177 (104.5825, -365.2789) -> (105.1903, -365.0271) projected
  line L178 (105.1903, -365.0271) -> (105.8425, -364.9413) projected
  line L179 (105.8425, -364.9413) -> (106.4947, -365.0271) projected
  line L180 (106.4947, -365.0271) -> (107.1025, -365.2789) projected
  line L181 (107.1025, -365.2789) -> (107.6244, -365.6794) projected
  line L182 (107.6244, -365.6794) -> (108.0249, -366.2013) projected
  line L183 (108.0249, -366.2013) -> (108.2766, -366.8091) projected
  line L184 (108.2766, -366.8091) -> (108.3625, -367.4613) projected
  line L185 (108.3625, -367.4613) -> (108.2766, -368.1135) projected
  line L186 (108.2766, -368.1135) -> (108.0249, -368.7213) projected
  line L187 (108.0249, -368.7213) -> (107.6244, -369.2432) projected
  line L188 (107.6244, -369.2432) -> (107.1025, -369.6437) projected
  line L189 (107.1025, -369.6437) -> (106.4947, -369.8954) projected
  line L190 (106.4947, -369.8954) -> (105.8425, -369.9813) projected
  line L191 (105.8425, -369.9813) -> (105.1903, -369.8954) projected
  line L192 (106.4947, -295.0271) -> (107.1025, -295.2789) projected
  line L193 (107.1025, -295.2789) -> (107.6244, -295.6793) projected
  line L194 (107.6244, -295.6793) -> (108.0249, -296.2012) projected
  line L195 (108.0249, -296.2012) -> (108.2766, -296.809) projected
  line L196 (108.2766, -296.809) -> (108.3625, -297.4613) projected
  line L197 (108.3625, -297.4613) -> (108.2766, -298.1135) projected
  line L198 (108.2766, -298.1135) -> (108.0249, -298.7212) projected
  line L199 (108.0249, -298.7212) -> (107.6244, -299.2432) projected
  line L200 (107.6244, -299.2432) -> (107.1025, -299.6437) projected
  line L201 (107.1025, -299.6437) -> (106.4947, -299.8954) projected
  line L202 (106.4947, -299.8954) -> (105.8425, -299.9813) projected
  line L203 (105.8425, -299.9813) -> (105.1903, -299.8954) projected
  line L204 (105.1903, -299.8954) -> (104.5825, -299.6437) projected
  line L205 (104.5825, -299.6437) -> (104.0606, -299.2432) projected
  line L206 (104.0606, -299.2432) -> (103.6601, -298.7212) projected
  line L207 (103.6601, -298.7212) -> (103.4084, -298.1135) projected
  line L208 (103.4084, -298.1135) -> (103.3225, -297.4613) projected
  line L209 (103.3225, -297.4613) -> (103.4084, -296.809) projected
  line L210 (103.4084, -296.809) -> (103.6601, -296.2012) projected
  line L211 (103.6601, -296.2012) -> (104.0606, -295.6793) projected
  line L212 (104.0606, -295.6793) -> (104.5825, -295.2789) projected
  line L213 (104.5825, -295.2789) -> (105.1903, -295.0271) projected
  line L214 (105.1903, -295.0271) -> (105.8425, -294.9413) projected
  line L215 (105.8425, -294.9413) -> (106.4947, -295.0271) projected
  line L216 (678.6601, -423.7213) -> (678.4084, -423.1135) projected
  line L217 (678.4084, -423.1135) -> (678.3225, -422.4613) projected
  line L218 (678.3225, -422.4613) -> (678.4084, -421.8091) projected
  line L219 (678.4084, -421.8091) -> (678.6601, -421.2013) projected
  line L220 (678.6601, -421.2013) -> (679.0606, -420.6794) projected
  line L221 (679.0606, -420.6794) -> (679.5825, -420.2789) projected
  line L222 (679.5825, -420.2789) -> (680.1903, -420.0271) projected
  line L223 (680.1903, -420.0271) -> (680.8425, -419.9413) projected
  line L224 (680.8425, -419.9413) -> (681.4947, -420.0271) projected
  line L225 (681.4947, -420.0271) -> (682.1025, -420.2789) projected
  line L226 (682.1025, -420.2789) -> (682.6244, -420.6794) projected
  line L227 (682.6244, -420.6794) -> (683.0249, -421.2013) projected
  line L228 (683.0249, -421.2013) -> (683.2766, -421.8091) projected
  line L229 (683.2766, -421.8091) -> (683.3625, -422.4613) projected
  line L230 (683.3625, -422.4613) -> (683.2766, -423.1135) projected
  line L231 (683.2766, -423.1135) -> (683.0249, -423.7213) projected
  line L232 (683.0249, -423.7213) -> (682.6244, -424.2432) projected
  line L233 (682.6244, -424.2432) -> (682.1025, -424.6437) projected
  line L234 (682.1025, -424.6437) -> (681.4947, -424.8954) projected
  line L235 (681.4947, -424.8954) -> (680.8425, -424.9813) projected
  line L236 (680.8425, -424.9813) -> (680.1903, -424.8954) projected
  line L237 (680.1903, -424.8954) -> (679.5825, -424.6437) projected
  line L238 (679.5825, -424.6437) -> (679.0606, -424.2432) projected
  line L239 (679.0606, -424.2432) -> (678.6601, -423.7213) projected
  line L240 (623.6601, -368.7213) -> (623.4084, -368.1135) projected
  line L241 (623.4084, -368.1135) -> (623.3225, -367.4613) projected
  line L242 (623.3225, -367.4613) -> (623.4084, -366.8091) projected
  line L243 (623.4084, -366.8091) -> (623.6601, -366.2013) projected
  line L244 (623.6601, -366.2013) -> (624.0606, -365.6794) projected
  line L245 (624.0606, -365.6794) -> (624.5825, -365.2789) projected
  line L246 (624.5825, -365.2789) -> (625.1903, -365.0271) projected
  line L247 (625.1903, -365.0271) -> (625.8425, -364.9413) projected
  line L248 (625.8425, -364.9413) -> (626.4947, -365.0271) projected
  line L249 (626.4947, -365.0271) -> (627.1025, -365.2789) projected
  line L250 (627.1025, -365.2789) -> (627.6244, -365.6794) projected
  line L251 (627.6244, -365.6794) -> (628.0249, -366.2013) projected
  line L252 (628.0249, -366.2013) -> (628.2766, -366.8091) projected
  line L253 (628.2766, -366.8091) -> (628.3625, -367.4613) projected
  line L254 (628.3625, -367.4613) -> (628.2766, -368.1135) projected
  line L255 (628.2766, -368.1135) -> (628.0249, -368.7213) projected
  line L256 (628.0249, -368.7213) -> (627.6244, -369.2432) projected
  line L257 (627.6244, -369.2432) -> (627.1025, -369.6437) projected
  line L258 (627.1025, -369.6437) -> (626.4947, -369.8954) projected
  line L259 (626.4947, -369.8954) -> (625.8425, -369.9813) projected
  line L260 (625.8425, -369.9813) -> (625.1903, -369.8954) projected
  line L261 (625.1903, -369.8954) -> (624.5825, -369.6437) projected
  line L262 (624.5825, -369.6437) -> (624.0606, -369.2432) projected
  line L263 (624.0606, -369.2432) -> (623.6601, -368.7213) projected
  line L264 (623.6601, -298.7212) -> (623.4084, -298.1135) projected
  line L265 (623.4084, -298.1135) -> (623.3225, -297.4613) projected
  line L266 (623.3225, -297.4613) -> (623.4084, -296.809) projected
  line L267 (623.4084, -296.809) -> (623.6601, -296.2012) projected
  line L268 (623.6601, -296.2012) -> (624.0606, -295.6793) projected
  line L269 (624.0606, -295.6793) -> (624.5825, -295.2789) projected
  line L270 (624.5825, -295.2789) -> (625.1903, -295.0271) projected
  line L271 (625.1903, -295.0271) -> (625.8425, -294.9413) projected
  line L272 (625.8425, -294.9413) -> (626.4947, -295.0271) projected
  line L273 (626.4947, -295.0271) -> (627.1025, -295.2789) projected
  line L274 (627.1025, -295.2789) -> (627.6244, -295.6793) projected
  line L275 (627.6244, -295.6793) -> (628.0249, -296.2012) projected
  line L276 (628.0249, -296.2012) -> (628.2766, -296.809) projected
  line L277 (628.2766, -296.809) -> (628.3625, -297.4613) projected
  line L278 (628.3625, -297.4613) -> (628.2766, -298.1135) projected
  line L279 (628.2766, -298.1135) -> (628.0249, -298.7212) projected
  line L280 (628.0249, -298.7212) -> (627.6244, -299.2432) projected
  line L281 (627.6244, -299.2432) -> (627.1025, -299.6437) projected
  line L282 (627.1025, -299.6437) -> (626.4947, -299.8954) projected
  line L283 (626.4947, -299.8954) -> (625.8425, -299.9813) projected
  line L284 (625.8425, -299.9813) -> (625.1903, -299.8954) projected
  line L285 (625.1903, -299.8954) -> (624.5825, -299.6437) projected
  line L286 (624.5825, -299.6437) -> (624.0606, -299.2432) projected
  line L287 (624.0606, -299.2432) -> (623.6601, -298.7212) projected
  line L288 (678.6601, -368.7213) -> (678.4084, -368.1135) projected
  line L289 (678.4084, -368.1135) -> (678.3225, -367.4613) projected
  line L290 (678.3225, -367.4613) -> (678.4084, -366.8091) projected
  line L291 (678.4084, -366.8091) -> (678.6601, -366.2013) projected
  line L292 (678.6601, -366.2013) -> (679.0606, -365.6794) projected
  line L293 (679.0606, -365.6794) -> (679.5825, -365.2789) projected
  line L294 (679.5825, -365.2789) -> (680.1903, -365.0271) projected
  line L295 (680.1903, -365.0271) -> (680.8425, -364.9413) projected
  line L296 (680.8425, -364.9413) -> (681.4947, -365.0271) projected
  line L297 (681.4947, -365.0271) -> (682.1025, -365.2789) projected
  line L298 (682.1025, -365.2789) -> (682.6244, -365.6794) projected
  line L299 (682.6244, -365.6794) -> (683.0249, -366.2013) projected
  line L300 (683.0249, -366.2013) -> (683.2766, -366.8091) projected
  line L301 (683.2766, -366.8091) -> (683.3625, -367.4613) projected
  line L302 (683.3625, -367.4613) -> (683.2766, -368.1135) projected
  line L303 (683.2766, -368.1135) -> (683.0249, -368.7213) projected
  line L304 (683.0249, -368.7213) -> (682.6244, -369.2432) projected
  line L305 (682.6244, -369.2432) -> (682.1025, -369.6437) projected
  line L306 (682.1025, -369.6437) -> (681.4947, -369.8954) projected
  line L307 (681.4947, -369.8954) -> (680.8425, -369.9813) projected
  line L308 (680.8425, -369.9813) -> (680.1903, -369.8954) projected
  line L309 (680.1903, -369.8954) -> (679.5825, -369.6437) projected
  line L310 (679.5825, -369.6437) -> (679.0606, -369.2432) projected
  line L311 (679.0606, -369.2432) -> (678.6601, -368.7213) projected
  line L312 (678.6601, -296.2012) -> (679.0606, -295.6793) projected
  line L313 (679.0606, -295.6793) -> (679.5825, -295.2789) projected
  line L314 (679.5825, -295.2789) -> (680.1903, -295.0271) projected
  line L315 (680.1903, -295.0271) -> (680.8425, -294.9413) projected
  line L316 (680.8425, -294.9413) -> (681.4947, -295.0271) projected
  line L317 (681.4947, -295.0271) -> (682.1025, -295.2789) projected
  line L318 (682.1025, -295.2789) -> (682.6244, -295.6793) projected
  line L319 (682.6244, -295.6793) -> (683.0249, -296.2012) projected
  line L320 (683.0249, -296.2012) -> (683.2766, -296.809) projected
  line L321 (683.2766, -296.809) -> (683.3625, -297.4613) projected
  line L322 (683.3625, -297.4613) -> (683.2766, -298.1135) projected
  line L323 (683.2766, -298.1135) -> (683.0249, -298.7212) projected
  line L324 (683.0249, -298.7212) -> (682.6244, -299.2432) projected
  line L325 (682.6244, -299.2432) -> (682.1025, -299.6437) projected
  line L326 (682.1025, -299.6437) -> (681.4947, -299.8954) projected
  line L327 (681.4947, -299.8954) -> (680.8425, -299.9813) projected
  line L328 (680.8425, -299.9813) -> (680.1903, -299.8954) projected
  line L329 (680.1903, -299.8954) -> (679.5825, -299.6437) projected
  line L330 (679.5825, -299.6437) -> (679.0606, -299.2432) projected
  line L331 (679.0606, -299.2432) -> (678.6601, -298.7212) projected
  line L332 (678.6601, -298.7212) -> (678.4084, -298.1135) projected
  line L333 (678.4084, -298.1135) -> (678.3225, -297.4613) projected
  line L334 (678.3225, -297.4613) -> (678.4084, -296.809) projected
  line L335 (678.4084, -296.809) -> (678.6601, -296.2012) projected
  line L336 (363.6601, -368.7213) -> (363.4084, -368.1135) projected
  line L337 (363.4084, -368.1135) -> (363.3225, -367.4613) projected
  line L338 (363.3225, -367.4613) -> (363.4084, -366.8091) projected
  line L339 (363.4084, -366.8091) -> (363.6601, -366.2013) projected
  line L340 (363.6601, -366.2013) -> (364.0606, -365.6794) projected
  line L341 (364.0606, -365.6794) -> (364.5825, -365.2789) projected
  line L342 (364.5825, -365.2789) -> (365.1903, -365.0271) projected
  line L343 (365.1903, -365.0271) -> (365.8425, -364.9413) projected
  line L344 (365.8425, -364.9413) -> (366.4947, -365.0271) projected
  line L345 (366.4947, -365.0271) -> (367.1025, -365.2789) projected
  line L346 (367.1025, -365.2789) -> (367.6244, -365.6794) projected
  line L347 (367.6244, -365.6794) -> (368.0249, -366.2013) projected
  line L348 (368.0249, -366.2013) -> (368.2766, -366.8091) projected
  line L349 (368.2766, -366.8091) -> (368.3625, -367.4613) projected
  line L350 (368.3625, -367.4613) -> (368.2766, -368.1135) projected
  line L351 (368.2766, -368.1135) -> (368.0249, -368.7213) projected
  line L352 (368.0249, -368.7213) -> (367.6244, -369.2432) projected
  line L353 (367.6244, -369.2432) -> (367.1025, -369.6437) projected
  line L354 (367.1025, -369.6437) -> (366.4947, -369.8954) projected
  line L355 (366.4947, -369.8954) -> (365.8425, -369.9813) projected
  line L356 (365.8425, -369.9813) -> (365.1903, -369.8954) projected
  line L357 (365.1903, -369.8954) -> (364.5825, -369.6437) projected
  line L358 (364.5825, -369.6437) -> (364.0606, -369.2432) projected
  line L359 (364.0606, -369.2432) -> (363.6601, -368.7213) projected
  line L360 (363.6601, -298.7212) -> (363.4084, -298.1135) projected
  line L361 (363.4084, -298.1135) -> (363.3225, -297.4613) projected
  line L362 (363.3225, -297.4613) -> (363.4084, -296.809) projected
  line L363 (363.4084, -296.809) -> (363.6601, -296.2012) projected
  line L364 (363.6601, -296.2012) -> (364.0606, -295.6793) projected
  line L365 (364.0606, -295.6793) -> (364.5825, -295.2789) projected
  line L366 (364.5825, -295.2789) -> (365.1903, -295.0271) projected
  line L367 (365.1903, -295.0271) -> (365.8425, -294.9413) projected
  line L368 (365.8425, -294.9413) -> (366.4947, -295.0271) projected
  line L369 (366.4947, -295.0271) -> (367.1025, -295.2789) projected
  line L370 (367.1025, -295.2789) -> (367.6244, -295.6793) projected
  line L371 (367.6244, -295.6793) -> (368.0249, -296.2012) projected
  line L372 (368.0249, -296.2012) -> (368.2766, -296.809) projected
  line L373 (368.2766, -296.809) -> (368.3625, -297.4613) projected
  line L374 (368.3625, -297.4613) -> (368.2766, -298.1135) projected
  line L375 (368.2766, -298.1135) -> (368.0249, -298.7212) projected
  line L376 (368.0249, -298.7212) -> (367.6244, -299.2432) projected
  line L377 (367.6244, -299.2432) -> (367.1025, -299.6437) projected
  line L378 (367.1025, -299.6437) -> (366.4947, -299.8954) projected
  line L379 (366.4947, -299.8954) -> (365.8425, -299.9813) projected
  line L380 (365.8425, -299.9813) -> (365.1903, -299.8954) projected
  line L381 (365.1903, -299.8954) -> (364.5825, -299.6437) projected
  line L382 (364.5825, -299.6437) -> (364.0606, -299.2432) projected
  line L383 (364.0606, -299.2432) -> (363.6601, -298.7212) projected
  line L384 (35.8425, -283.4613) -> (695.8425, -283.4613) projected
  line L385 (35.8425, -447.4613) -> (35.8425, -283.4613) projected
  line L386 (35.8823, -447.8653) -> (35.8425, -447.4613) projected
  line L387 (36.0002, -448.2538) -> (35.8823, -447.8653) projected
  line L388 (36.1915, -448.6119) -> (36.0002, -448.2538) projected
  line L389 (36.4491, -448.9257) -> (36.1915, -448.6119) projected
  line L390 (36.7629, -449.1833) -> (36.4491, -448.9257) projected
  line L391 (37.121, -449.3747) -> (36.7629, -449.1833) projected
  line L392 (37.5095, -449.4925) -> (37.121, -449.3747) projected
  line L393 (37.9136, -449.5323) -> (37.5095, -449.4925) projected
  line L394 (38.3176, -449.4925) -> (37.9136, -449.5323) projected
  line L395 (38.7061, -449.3747) -> (38.3176, -449.4925) projected
  line L396 (39.0642, -449.1833) -> (38.7061, -449.3747) projected
  line L397 (39.378, -448.9257) -> (39.0642, -449.1833) projected
  line L398 (105.8425, -382.4613) -> (39.378, -448.9257) projected
  line L399 (625.8425, -382.4613) -> (105.8425, -382.4613) projected
  line L400 (692.307, -448.9257) -> (625.8425, -382.4613) projected
  line L401 (692.6208, -449.1833) -> (692.307, -448.9257) projected
  line L402 (692.9789, -449.3747) -> (692.6208, -449.1833) projected
  line L403 (693.3674, -449.4925) -> (692.9789, -449.3747) projected
  line L404 (693.7714, -449.5323) -> (693.3674, -449.4925) projected
  line L405 (694.1755, -449.4925) -> (693.7714, -449.5323) projected
  line L406 (694.564, -449.3747) -> (694.1755, -449.4925) projected
  line L407 (694.9221, -449.1833) -> (694.564, -449.3747) projected
  line L408 (695.2359, -448.9257) -> (694.9221, -449.1833) projected
  line L409 (695.4935, -448.6119) -> (695.2359, -448.9257) projected
  line L410 (695.6848, -448.2538) -> (695.4935, -448.6119) projected
  line L411 (695.8027, -447.8653) -> (695.6848, -448.2538) projected
  line L412 (695.8425, -447.4613) -> (695.8027, -447.8653) projected
  line L413 (695.8425, -283.4613) -> (695.8425, -447.4613) projected
  circle A0 centre (680.8425, -422.4613) radius 2.4984
  circle A1 centre (625.8425, -297.4613) radius 2.4984
  circle A2 centre (494.7925, -297.4613) radius 2.4984
  circle A3 centre (494.7925, -367.4613) radius 2.4985
  circle A4 centre (365.8425, -367.4613) radius 2.4984
  circle A5 centre (365.8425, -297.4613) radius 2.4984
  circle A6 centre (236.8925, -297.4612) radius 2.4985
  circle A7 centre (236.8925, -367.4613) radius 2.4984
  circle A8 centre (105.8425, -367.4613) radius 2.4984
  circle A9 centre (50.8425, -367.4613) radius 2.4984
  circle A10 centre (50.8425, -422.4613) radius 2.4984
  circle A11 centre (50.8425, -297.4613) radius 2.4984
  circle A12 centre (105.8425, -297.4613) radius 2.4984
  circle A13 centre (625.8425, -367.4613) radius 2.4984
  circle A14 centre (680.8425, -367.4613) radius 2.4984
  circle A15 centre (680.8425, -297.4613) radius 2.4984
  point P0 (-87.4375, -600)
  constraints: 48 tangent, 16 centre point
hole "Hole1" at (768.28, 177.5387, -660) at (768.28, 232.5387, -660) at (713.28, 232.5387, -660) at (768.28, 302.5387, -660) at (713.28, 302.5387, -660) at (582.23, 232.5387, -660) at (582.23, 302.5387, -660) at (453.28, 302.5387, -660) at (453.28, 232.5387, -660) at (324.33, 232.5387, -660) at (324.33, 302.5388, -660) at (193.28, 302.5387, -660) at (193.28, 232.5387, -660) at (138.28, 232.5387, -660) at (138.28, 302.5387, -660) at (138.28, 177.5387, -660) direction (0, 0, -1) diameter 5.2 end through all
body "Solid1"
